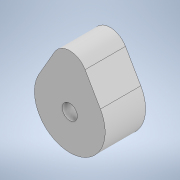
# Autodesk Inventor part: Pear cam 2
Saved by Autodesk Inventor 2021 (Build 250183000, 183)
## iProperties
Created: 2021-04-11
Part Number: Pear cam 2
Material: Generic
Document SubType Name: Modeling
Designer: Nabeel Azafer
Density: 1 g/cm^3
Appearance: Default
Author: Nabeel Azafer
Autodesk Inventor part; units mm, degrees
ref_plane "YZ Plane" through (0, 0, 0) normal (1, 0, 0) x (0, 1, 0)
ref_plane "XZ Plane" through (0, 0, 0) normal (0, 1, 0) x (-1, 0, 0)
ref_plane "XY Plane" through (0, 0, 0) normal (0, 0, 1) x (1, 0, 0)
sketch "Sketch5" plane through (0, 0, 0) normal (0, 0, 1) x (1, 0, 0)
  arc A0 (-6.0622, 3.5) -> (6.0622, 3.5) centre (0, 0) ccw
  arc A1 (3.0311, 8.75) -> (-3.0311, 8.75) centre (0, 7) ccw
  line L0 (-6.0622, 3.5) -> (-3.0311, 8.75)
  line L1 (3.0311, 8.75) -> (6.0622, 3.5)
  circle A2 centre (0, 0) radius 1.5
  dimension "d21" = 14
  dimension "d22" = 7
  dimension "d23" = 7
  dimension "d24" = 3
  constraints: 4 end point, 4 point on circle, 4 tangent, 3 centre point, 2 coincident, 1 vertical alignment
  measures "d21" diameter of A0
  measures "d22" diameter of A1
  measures "d23" distance of point (0, 0) A1.centre
  measures "d24" diameter of A2
extrude "Extrusion3" add sketch "Sketch5" along normal blind 8
body "Solid2"
